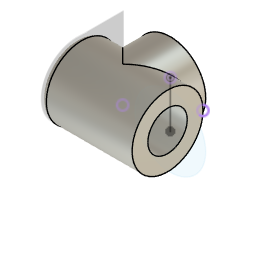
Link6 v11 (Autodesk Fusion 360 design; units mm, degrees)
Autodesk Fusion 360 part; units mm, degrees
sketch "Boceto1" plane through (0, 0, 0) normal (1, 0, 0) x (0, 0, -1)
  circle A0 centre (0, 0) radius 45
  dimension "d1" = 90
  constraint coincident A0.centre origin
  measures "d1" diameter of A0
extrude "Extruir1" add sketch "Boceto1" along normal blind 60.5
sketch "Boceto2" plane through (0, 0, 0) normal (0, 0, 1) x (1, 0, 0)
  circle A0 centre (60.5, 0) radius 45
  line L0 (0, -45) -> (0, 45)
  dimension "d4" = 90
  dimension "d5" = 60.5
  measures "d4" diameter of A0
  measures "d5" distance of A0.centre L0
extrude "Extruir2" add sketch "Boceto2" along normal blind 57 and the other way blind 59
sketch "Boceto3" plane through (0, 0, -59) normal (0, 0, -1) x (-1, 0, 0)
  circle A0 centre (-60.5, 0) radius 45
  circle A1 centre (-60.5, 0) radius 25
  dimension "d10" = 50
  constraint concentric A0 A1
  measures "d10" diameter of A1
extrude "Extruir3" cut sketch "Boceto3" along normal through all and the other way through all contours A1
fillet "Empalme1" radius 7 1 edges at (18.5453, 16.2727, -59)
move_body "Desplazar1" bodies 1 to x (1, 0, 0) y (0, 0, -1) z (0, 1, 0) at (0, 59, -59)
move_body "Desplazar2" bodies 1 to x (1, 0, 0) y (0, 1, 0) z (0, 0, 1) at (0, -13.9982, -0.2247)
sketch "Sketch4" plane through (0, 0, 0) normal (0, 0, 1) x (1, 0, 0)
move_body "Move3" bodies 1 to x (1, 0, 0) y (0, 1, 0) z (0, 0, 1) at (0, -45, 0)
sketch "Sketch5" plane through (0, 0, 0) normal (-1, 0, 0) x (0, 0, 1)
  circle A0 centre (-59.2247, 0.0018) radius 45
  line L0 (-59.2247, 0.0018) -> (0, 0)
  dimension "d15" = 59.2247
  constraint coincident A0.centre L0.start
  constraint coincident L0.end origin
  measures "d15" horizontal distance of L0.end A0.centre
move_body "Move4" bodies 1 to x (1, 0, 0) y (0, 1, 0) z (0, 0, 1) at (0, 0, 59.225)
sketch "Sketch6" plane through (0, 0, 0) normal (0, 0, 1) x (1, 0, 0)
  point P0 (60.5, 0.0018)
  point P1 (15.5, 57.0018)
  dimension "d16" = 60.5
  dimension "d17" = 57.0018
  measures "d16" horizontal distance of P0 origin
  measures "d17" vertical distance of origin P1
sketch "Sketch7" plane through (0, 0, 0) normal (0, 0, 1) x (1, 0, 0)
